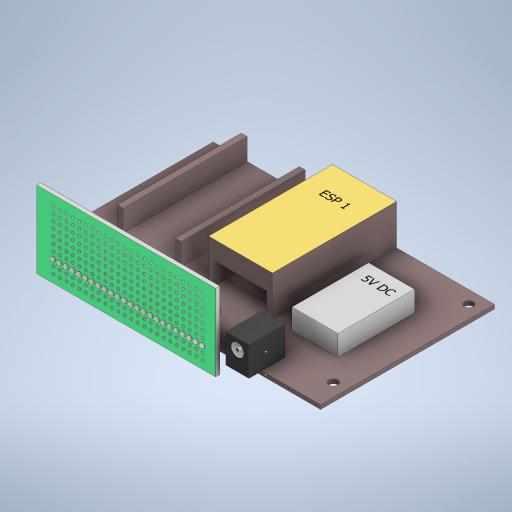
# Autodesk Inventor part: pcb_main_populated
Saved by Autodesk Inventor 2023 (Build 270158000, 158)
## iProperties
Created: 2023-05-16
Part Number: pcb_main_populated
Material: Generic
Document SubType Name: Modeling
Designer: mark
Density: 1 g/cm^3
Appearance: Default
Author: mark
Autodesk Inventor part; units mm, degrees
ref_plane "YZ Plane" through (0, 0, 0) normal (1, 0, 0) x (0, 1, 0)
ref_plane "XZ Plane" through (0, 0, 0) normal (0, 1, 0) x (-1, 0, 0)
ref_plane "XY Plane" through (0, 0, 0) normal (0, 0, 1) x (1, 0, 0)
sketch "Sketch1" plane through (0, 0, 0) normal (0, 1, 0) x (-1, 0, 0)
  line L0 (97.0183, -76.5155) -> (-12.9817, -76.5155)
  line L1 (-12.9817, -76.5155) -> (-12.9817, -8.5155)
  line L2 (-12.9817, -8.5155) -> (97.0183, -8.5155)
  line L3 (97.0183, -8.5155) -> (97.0183, -76.5155)
  circle A0 centre (92.0183, -71.5155) radius 1.75
  circle A1 centre (-7.9817, -71.5155) radius 1.75
  circle A2 centre (92.0183, -18.5155) radius 1.75
  circle A3 centre (-7.9817, -18.5155) radius 1.75
  point P0 (0, 0)
  dimension "d0" = 110
  dimension "d1" = 68
  dimension "d2" = 3.5
  dimension "d3" = 3.5
  dimension "d4" = 5
  dimension "d5" = 5
  dimension "d6" = 5
  dimension "d7" = 5
  dimension "d8" = 3.5
  dimension "d9" = 3.5
  dimension "d10" = 53
  dimension "d11" = 53
  dimension "d12" = 5
  dimension "d13" = 5
  constraints: 8 end point, 4 centre point, 2 parallel, 1 horizontal, 1 perpendicular
  measures "d0" distance of L1.end L2.end
  measures "d1" distance of L0.end L1.end
  measures "d2" diameter of A0
  measures "d3" diameter of A1
  measures "d4" distance from line of L0 A0.centre
  measures "d5" distance from line of L3 A0.centre
  measures "d6" distance from line of L1 A1.centre
  measures "d7" distance from line of L0 A1.centre
  measures "d8" diameter of A2
  measures "d9" diameter of A3
  measures "d10" distance of A1.centre A3.centre
  measures "d11" distance of A2.centre A0.centre
  measures "d12" distance from line of L3 A2.centre
  measures "d13" distance from line of L1 A3.centre
extrude "Extrusion1" add sketch "Sketch1" along normal blind 1.6
sketch "Sketch2" plane through (0, 1.6, 0) normal (0, 1, 0) x (1, 0, 0)
  line L0 (12.9817, 76.5155) -> (-97.0183, 76.5155) projected
  line L1 (-86.0183, 76.5155) -> (-83.7183, 76.5155)
  line L2 (-83.7183, 76.5155) -> (-83.7183, 28.0155)
  line L3 (-83.7183, 28.0155) -> (-86.0183, 28.0155)
  line L4 (-86.0183, 28.0155) -> (-86.0183, 76.5155)
  line L5 (-97.0183, 76.5155) -> (-97.0183, 8.5155) projected
  line L6 (-61.0183, 76.5155) -> (-61.0183, 28.0155)
  line L7 (-61.0183, 28.0155) -> (-63.3183, 28.0155)
  line L8 (-63.3183, 28.0155) -> (-63.3183, 76.5155)
  line L9 (-63.3183, 76.5155) -> (-61.0183, 76.5155)
  line L10 (-50.3183, 76.5155) -> (-48.0183, 76.5155)
  line L11 (-48.0183, 76.5155) -> (-48.0183, 28.0155)
  line L12 (-48.0183, 28.0155) -> (-50.3183, 28.0155)
  line L13 (-50.3183, 28.0155) -> (-50.3183, 76.5155)
  line L14 (-25.3183, 76.5155) -> (-25.3183, 28.0155)
  line L15 (-25.3183, 28.0155) -> (-27.6183, 28.0155)
  line L16 (-27.6183, 28.0155) -> (-27.6183, 76.5155)
  line L17 (-27.6183, 76.5155) -> (-25.3183, 76.5155)
  point P0 (0, 0)
  dimension "d16" = 2.3
  dimension "d17" = 48.5
  dimension "d18" = 11
  dimension "d21" = 22.7
  dimension "d28" = 35.7
  constraints: 32 end point, 3 horizontal, 2 parallel, 1 perpendicular, 1 point on line, 24 other
  measures "d16" distance of L2.end L3.end
  measures "d17" distance of L1.end L2.end
  measures "d18" distance between parallel lines of L5 L4
  measures "d21" distance of L1.end L6.start
  measures "d28" distance of L1.start L10.start
extrude "Extrusion2" add sketch "Sketch2" along normal blind 8.5
sketch "Sketch3" plane through (0, 1.6, 0) normal (0, 1, 0) x (1, 0, 0)
  line L0 (-97.0183, 8.5155) -> (12.9817, 8.5155) projected
  line L1 (-88.7183, 8.5155) -> (-37.2183, 8.5155)
  line L2 (-37.2183, 8.5155) -> (-37.2183, 19.5155)
  line L3 (-37.2183, 19.5155) -> (-88.7183, 19.5155)
  line L4 (-88.7183, 19.5155) -> (-88.7183, 8.5155)
  line L5 (-97.0183, 76.5155) -> (-97.0183, 8.5155) projected
  point P0 (0, 0)
  point P1 (-88.7183, 14.0155)
  dimension "d35" = 51.5
  dimension "d36" = 11
  dimension "d37" = 8.3
  constraints: 8 end point, 2 parallel, 1 horizontal, 1 midpoint, 1 perpendicular, 1 point on line
  measures "d35" distance of L3.end L2.end
  measures "d36" distance of L2.end L1.end
  measures "d37" distance from line of L5 point (-88.718, 14.016)
extrude "Extrusion3" add sketch "Sketch3" along normal blind 2.5
sketch "Sketch4" plane through (0, 10.1, 0) normal (0, 1, 0) x (1, 0, 0)
  line L0 (12.9817, 76.5155) -> (-25.3183, 76.5155) projected
  line L1 (-48.0183, 28.0155) -> (-50.3183, 28.0155) projected
  line L2 (-25.3183, 76.5155) -> (-50.3183, 76.5155)
  line L3 (-50.3183, 76.5155) -> (-50.3183, 28.0155)
  line L4 (-50.3183, 28.0155) -> (-25.3183, 28.0155)
  line L5 (-25.3183, 28.0155) -> (-25.3183, 76.5155)
  point P0 (0, 0)
  constraints: 8 end point, 2 parallel, 1 horizontal, 1 perpendicular
extrude "Extrusion4" add sketch "Sketch4" along normal blind 7.2
sketch "Sketch5" plane through (0, 17.3, 0) normal (0, 1, 0) x (1, 0, 0)
  line L0 (-43.1805, 66.7123) -> (-30.878, 66.7123) construction
  line L1 (-30.878, 66.7123) -> (-30.878, 62.0023) construction
  line L2 (-30.878, 62.0023) -> (-43.1805, 62.0023) construction
  line L3 (-43.1805, 62.0023) -> (-43.1805, 66.7123) construction
  point P0 (0, 0)
  constraints: 2 other
sketch "Sketch6" plane through (-97.0183, 0, -8.5155) normal (0, 0, 1) x (1, 0, 0)
  line L0 (8.3, 1.6) -> (8.3, 4.1) projected
  line L1 (8.3, 4.1) -> (59.8, 4.1)
  line L2 (59.8, 4.1) -> (59.8, 1.6)
  line L3 (59.8, 1.6) -> (8.3, 1.6)
  line L4 (8.3, 1.6) -> (8.3, 4.1)
  point P0 (97.0183, 0)
  constraints: 8 end point, 2 parallel, 1 horizontal, 1 perpendicular
extrude "Extrusion5" add sketch "Sketch6" along normal blind 2.5
sketch "Sketch7" plane through (-97.0183, 0, -6.0155) normal (0, 0, 1) x (1, 0, 0)
  line L0 (3.1, 24.6) -> (73.1, 24.6)
  line L1 (73.1, 24.6) -> (73.1, -5.4)
  line L2 (73.1, -5.4) -> (3.1, -5.4)
  line L3 (3.1, -5.4) -> (3.1, 24.6)
  line L4 (59.8, 4.1) -> (8.3, 4.1) projected
  line L5 (8.3, 4.1) -> (8.3, 1.6) projected
  point P0 (97.0183, 0)
  point P1 (8.3, 2.85)
  dimension "d44" = 70
  dimension "d45" = 30
  dimension "d46" = 20.5
  dimension "d47" = 5.2
  constraints: 8 end point, 2 parallel, 1 horizontal, 1 midpoint, 1 perpendicular
  measures "d44" distance of L1.end L2.end
  measures "d45" distance of L0.end L1.end
  measures "d46" distance between parallel lines of L4 L0
  measures "d47" distance from line of point (8.3, 2.85) L3
extrude "Extrusion6" add sketch "Sketch7" along normal blind 1.6
sketch "Sketch8" plane through (-97.0183, 0, -4.4155) normal (0, 0, 1) x (1, 0, 0)
  circle A0 centre (9.6, 20.6) radius 0.5
  line L0 (73.1, 24.6) -> (3.1, 24.6) projected
  line L1 (3.1, 24.6) -> (3.1, -5.4) projected
  point P0 (97.0183, 0)
  dimension "d50" = 4
  dimension "d51" = 6.5
  dimension "d52" = 1
  constraints: 1 centre point
  measures "d50" distance from line of L0 A0.centre
  measures "d51" distance from line of L1 A0.centre
  measures "d52" diameter of A0
extrude "Extrusion7" cut sketch "Sketch8" against normal blind 1.6
pattern_linear "Rectangular Pattern1" count 10 spacing 2.54 along (0, -1, 0) count 24 spacing 2.54 along (1, 0, 0) of "Extrusion7"
sketch "Sketch9" plane through (0, 1.6, 0) normal (0, 1, 0) x (1, 0, 0)
  line L0 (-18.9183, 3.4155) -> (-9.9183, 3.4155)
  line L1 (-9.9183, 3.4155) -> (-9.9183, 17.4155)
  line L2 (-9.9183, 17.4155) -> (-18.9183, 17.4155)
  line L3 (-18.9183, 17.4155) -> (-18.9183, 3.4155)
  line L4 (-37.2183, 8.5155) -> (12.9817, 8.5155) projected
  line L5 (-23.9183, 6.0155) -> (-23.9183, 4.4155) projected
  point P0 (0, 0)
  point P1 (-23.9183, 5.2155)
  dimension "d61" = 9
  dimension "d62" = 14
  dimension "d63" = 5.1
  dimension "d66" = 5
  constraints: 8 end point, 2 parallel, 1 horizontal, 1 midpoint, 1 perpendicular
  measures "d61" distance of L2.end L1.end
  measures "d62" distance of L1.end L0.end
  measures "d63" distance between parallel lines of L4 L0
  measures "d66" distance from line of point (-23.918, 5.216) L3
extrude "Extrusion8" add sketch "Sketch9" along normal blind 11.4
sketch "Sketch10" plane through (-18.9183, 1.6, -3.4155) normal (0, 0, 1) x (1, 0, 0)
  circle A0 centre (4.5, 7.4) radius 2.5
  circle A1 centre (4.5, 7.4) radius 0.5
  line L0 (0, 11.4) -> (9, 11.4) projected
  line L1 (0, 0) -> (0, 11.4) projected
  point P0 (18.9183, -1.6)
  point P1 (4.5, 11.4)
  dimension "d67" = 5
  dimension "d68" = 1
  dimension "d69" = 4
  dimension "d70" = 4.5
  constraints: 2 centre point, 1 coincident, 1 midpoint
  measures "d67" diameter of A0
  measures "d68" diameter of A1
  measures "d69" distance of point (4.5, 11.4) A0.centre
  measures "d70" distance from line of L1 A0.centre
extrude "Extrusion9" cut sketch "Sketch10" against normal blind 8
sketch "Sketch11" plane through (0, 1.6, 0) normal (0, 1, 0) x (1, 0, 0)
  line L0 (-17.7183, 28.0155) -> (0.2817, 28.0155)
  line L1 (0.2817, 28.0155) -> (0.2817, 58.0155)
  line L2 (0.2817, 58.0155) -> (-17.7183, 58.0155)
  line L3 (-17.7183, 58.0155) -> (-17.7183, 28.0155)
  line L4 (-25.3183, 28.0155) -> (-25.3183, 76.5155) projected
  line L5 (-50.3183, 28.0155) -> (-25.3183, 28.0155) projected
  point P0 (0, 0)
  dimension "d73" = 18
  dimension "d74" = 30
  dimension "d75" = 7.6
  constraints: 8 end point, 2 parallel, 1 collinear, 1 horizontal, 1 perpendicular
  measures "d73" distance of L2.end L1.end
  measures "d74" distance of L1.end L0.end
  measures "d75" distance between parallel lines of L4 L3
extrude "Extrusion10" add sketch "Sketch11" along normal blind 8
sketch "Sketch12" plane through (0, 9.6, 0) normal (0, 1, 0) x (1, 0, 0)
  line L0 (-13.8156, 53.7908) -> (-2.3572, 53.7908) construction
  line L1 (-2.3572, 53.7908) -> (-2.3572, 50.6242) construction
  line L2 (-2.3572, 50.6242) -> (-13.8156, 50.6242) construction
  line L3 (-13.8156, 50.6242) -> (-13.8156, 53.7908) construction
  point P0 (0, 0)
  constraints: 2 other
sketch "Sketch13" plane through (-97.0183, 0, -4.4155) normal (0, 0, 1) x (1, 0, 0)
  circle A0 centre (9.6, 2.82) radius 0.5 projected
  circle A1 centre (9.6, 2.82) radius 0.9
  point P0 (97.0183, 0)
  dimension "d78" = 1.8
  constraints: 1 centre point, 1 coincident
  measures "d78" diameter of A1
extrude "Extrusion11" add sketch "Sketch13" along normal blind 1.2 contours A0 | A1
chamfer "Chamfer1" distance 0.7 angle 55 1 edges at (-88.3183, 2.82, -3.2155) measured on face at (-87.1183, 2.5412, -3.2155)
pattern_linear "Rectangular Pattern2" count 24 spacing 2.54 along (1, 0, 0) of "Extrusion11", "Chamfer1"
equation "\"d3\" = d2"
equation "\"d8\" = d2"
equation "\"d9\" = d8"
equation "\"d11\" = d10"
equation "\"d12\" = d5"
equation "\"d13\" = d6"
body "Solid1"
